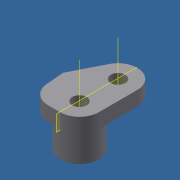
# Autodesk Inventor part: FingerTip_joint _v2
Saved by Autodesk Inventor 2014 SP2 (Build 180246200, 246)
## iProperties
Created: 2014-12-28
Part Number: FingerTip_joint _v2
Material: Generisch
Document SubType Name: Modeling
Designer: 4ndreas
Density: 1 g/cm^3
Appearance: Vorgabe
Mass: 0.472235 g
Surface Area: 6.54171 cm^2
Volume: 0.472235 cm^3
Author: 4ndreas
Autodesk Inventor part; units mm, degrees
ref_plane "YZ Plane" through (0, 0, 0) normal (1, 0, 0) x (0, 1, 0)
ref_plane "XZ Plane" through (0, 0, 0) normal (0, 1, 0) x (-1, 0, 0)
ref_plane "XY Plane" through (0, 0, 0) normal (0, 0, 1) x (1, 0, 0)
sketch "Skizze1" plane through (0, 0, 0) normal (0, 0, 1) x (1, 0, 0)
  circle A0 centre (0, 0) radius 4
  circle A1 centre (0, 8) radius 4
  line L0 (0, 0) -> (0, 8) construction
  line L1 (-4, 8) -> (-4, 0)
  line L2 (4, 0) -> (4, 8)
  dimension "d0" = 8
  dimension "d1" = 8
  dimension "d4" = 8
  constraints: 6 end point, 4 point on circle, 4 tangent, 2 centre point, 1 coincident, 1 vertical
  measures "d0" diameter of A0
  measures "d1" distance of L0.start L0.end
  measures "d4" diameter of A1
extrude "Extrusion1" add sketch "Skizze1" along normal blind 3
ref_plane "Arbeitsebene1" through (0, 8, 0) normal (1, 0, 0) x (0, 0, 1)
sketch "Skizze2" plane through (0, 0, 3) normal (0, 0, 1) x (1, 0, 0)
  arc A0 (-4, 0) -> (4, 0) centre (0, 0) ccw projected
  arc A1 (4, 8) -> (-4, 8) centre (0, 8) ccw projected
hole "Bohrung1" at (0, 8, 3) direction (0, 0, -1) diameter 3 end through all
hole "Bohrung2" at (0, 0, 3) direction (0, 0, -1) diameter 3 end through all
sketch "Skizze3" plane through (0, 0, 3) normal (0, 0, 1) x (1, 0, 0)
  arc A0 (-4, 0) -> (4, 0) centre (0, 0) ccw
  line L0 (4, 0) -> (4, 8)
  arc A1 (4, 8) -> (-4, 8) centre (0, 8) ccw
  line L1 (-6.5, 4) -> (-6.5, -4)
  line L2 (-6.5, -4) -> (0, -4)
  line L3 (-6.5, 4) -> (-3.570815, 9.802575)
  circle A2 centre (0, 0) radius 4 construction
  line L4 (0, 4) -> (-6.5, 4) construction
  circle A3 centre (0, 8) radius 1.5
  arc A4 (-4, 0) -> (4, 0) centre (0, 0) ccw
  circle A5 centre (0, 0) radius 1.5
  dimension "d16" = 6.5
  constraints: 10 end point, 6 point on circle, 3 coincident, 2 centre point, 2 tangent, 1 horizontal, 1 parallel, 1 perpendicular, 1 vertical alignment, 4 other
  measures "d16" distance from line of L1 point (0, 0)
extrude "Extrusion2" add sketch "Skizze3" against normal up to surface (3 mm away)
fillet "Rundung1" radius 4 1 edges at (-6.5, -4, 1.5)
sketch "Skizze4" plane through (0, 0, 0) normal (0, 0, -1) x (-1, 0, 0)
  arc A0 (-4, 0) -> (0, -4) centre (0, 0) ccw
  circle A1 centre (0, 0) radius 1.5
  circle A2 centre (0, 0) radius 4
  line L0 (6.5, 4) -> (0, 4)
  arc A3 (-4, 0) -> (0, -4) centre (0, 0) ccw projected
  circle A4 centre (0, 0) radius 1.5 projected
  point P0 (3.18396, 8.32)
  point P1 (3.97995, 0.4)
  constraints: 2 centre point, 2 coincident, 2 end point, 2 point on circle, 1 concentric, 1 horizontal, 1 vertical alignment, 4 other
sketch "Skizze4 outline for Extrusion3" plane through (0, 0, 0) normal (0, 0, -1) x (-1, 0, 0)
  circle A0 centre (0, 0) radius 4
  circle A1 centre (0, 0) radius 1.5
extrude "Extrusion3" add sketch "Skizze4 outline for Extrusion3" along normal blind 5.5
sketch "Skizze5" plane through (0, 0, 3) normal (0, 0, 1) x (1, 0, 0)
  arc A0 (-6.5, 0) -> (-2.5, -4) centre (-2.5, 0) ccw
  line L0 (-3.570815, 9.802575) -> (-6.5, 4)
  line L1 (-6.5, 4) -> (-6.5, 0)
  line L2 (-6.5, 4) -> (-6.811285, 3.383359)
  line L3 (-6.811285, 3.383359) -> (-6.484779, -0.348623)
  dimension "d26" = 5
  constraints: 4 end point, 1 collinear, 1 point on circle, 1 tangent
  measures "d26" angle of L3 L1
extrude "Extrusion4" add sketch "Skizze5" against normal up to surface (3 mm away)
equation "\"d0\" = Finger_diameter"
equation "\"d1\" = d0"
equation "\"d4\" = d0"
equation "\"d2\" = Join_width"
equation "\"d5\" = bearingHole"
equation "\"d19\" = bearingHole"
equation "\"FingerLaenge_B\" = 25"
equation "\"Hebel_B\" = 25"
equation "\"Finger_width\" = 22"
equation "\"Finger_diameter\" = 8"
equation "\"FingerWall\" = 3"
equation "\"Hebel_basis_2\" = 15"
equation "\"Join_width\" = 3"
equation "\"bearingHole\" = 3"
equation "\"bearingWall\" = 4"
equation "\"support_D\" = 0.25"
